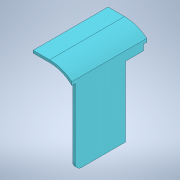
# Autodesk Inventor part: obudowa przekładni 3 LEFT
Saved by Autodesk Inventor 2021 (Build 250183000, 183)
## iProperties
Created: 2022-01-26
Part Number: obudowa przekładni 3 LEFT
Material: Generic
Document SubType Name: Modeling
Designer: Łukasz
Density: 1 g/cm^3
Appearance: Cadet Blue
Author: Łukasz
Autodesk Inventor part; units mm, degrees
ref_plane "YZ Plane" through (0, 0, 0) normal (1, 0, 0) x (0, 1, 0)
ref_plane "XZ Plane" through (0, 0, 0) normal (0, 1, 0) x (-1, 0, 0)
ref_plane "XY Plane" through (0, 0, 0) normal (0, 0, 1) x (1, 0, 0)
sketch "Sketch1" plane through (0, 0, 0) normal (0, 0, 1) x (1, 0, 0)
  arc A0 (136, 96.5127) -> (109, 107) centre (109, 67) ccw
  line L0 (149, 0) -> (149, 67)
  line L1 (109, 107) -> (89, 107)
  line L2 (149, 0) -> (136, 0)
  line L3 (136, 0) -> (136, 112.2002)
  line L4 (89, 110) -> (109, 110)
  arc A1 (136, 100.4664) -> (109, 110) centre (109, 67) ccw
  line L5 (89, 107) -> (89, 110)
  point P0 (0, 0)
  point P1 (0, 53.5)
  dimension "d0" = 13
  dimension "d1" = 3
  constraints: 12 end point, 4 point on circle, 2 centre point, 2 point on line, 1 horizontal, 1 perpendicular, 1 vertical
  measures "d0" distance of L0.start L2.end
  measures "d1" distance between parallel lines of L1 L4
extrude "Extrusion1" add sketch "Sketch1" along normal blind 91
sketch "Sketch2" plane through (136, 96.5127, 0) normal (1, 0, 0) x (0, 0, -1)
  line L0 (0, 3.9537) -> (-91, 3.9537) projected
  line L1 (-87, 3.9537) -> (-4, 3.9537)
  line L2 (-4, 3.9537) -> (-4, -92.0463)
  line L3 (-4, -92.0463) -> (-87, -92.0463)
  line L4 (-87, -92.0463) -> (-87, 3.9537)
  line L5 (-91, 0) -> (-91, 3.9537) projected
  point P0 (0, -96.5127)
  point P1 (-4, 3.9537)
  dimension "d4" = 83
  dimension "d5" = 96
  dimension "d6" = 4
  constraints: 8 end point, 2 parallel, 1 horizontal, 1 perpendicular, 1 point on line
  measures "d4" distance of L2.end L3.end
  measures "d5" distance of L1.end L2.end
  measures "d6" distance between parallel lines of L5 L4
extrude "Extrusion2" add sketch "Sketch2" against normal blind 3
fillet "Fillet1" radius 8 1 edges at (134.5, 4.4664, 87)
sketch "Sketch3" plane through (136, 96.5127, 0) normal (1, 0, 0) x (0, 0, -1)
  line L0 (-79, -92.0463) -> (-4, -92.0463) projected
  line L1 (-4, -92.0463) -> (-26, -92.0463)
  line L2 (-26, -92.0463) -> (-26, -7.0463)
  line L3 (-26, -7.0463) -> (-4, -7.0463)
  line L4 (-4, -7.0463) -> (-4, -92.0463)
  point P0 (0, -96.5127)
  dimension "d10" = 22
  dimension "d11" = 85
  constraints: 8 end point, 2 parallel, 1 horizontal, 1 perpendicular
  measures "d10" distance of L2.end L3.end
  measures "d11" distance of L1.end L2.end
extrude "Extrusion3" cut sketch "Sketch3" against normal up to surface (3 mm away)
body "Solid1"
